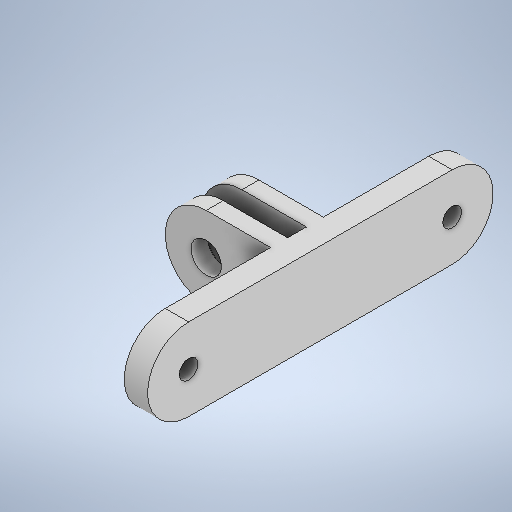
# Autodesk Inventor part: support_realsense
Saved by Autodesk Inventor 2025.2 (Build 292293000, 293)
## iProperties
Created: 2025-05-11
Part Number: support_realsense
Material: Générique
Document SubType Name: Modeling
Designer: enezl
Density: 1 g/cm^3
Appearance: Par défaut
Author: enezl
Autodesk Inventor part; units mm, degrees
ref_plane "YZ Plane" through (0, 0, 0) normal (1, 0, 0) x (0, 1, 0)
ref_plane "XZ Plane" through (0, 0, 0) normal (0, 1, 0) x (-1, 0, 0)
ref_plane "XY Plane" through (0, 0, 0) normal (0, 0, 1) x (1, 0, 0)
sketch "Esquisse1" plane through (0, 0, 0) normal (1, 0, 0) x (0, 1, 0)
  line L0 (0, 22.5) -> (0, -22.5) construction
  line L1 (-7, 22.5) -> (-7, -22.5)
  line L2 (7, -22.5) -> (7, 22.5)
  arc A0 (7, 22.5) -> (-7, 22.5) centre (0, 22.5) ccw
  arc A1 (-7, -22.5) -> (7, -22.5) centre (0, -22.5) ccw
  circle A2 centre (0, 22.5) radius 1.6
  circle A3 centre (0, -22.5) radius 1.6
  point P0 (0, 0)
  dimension "d0" = 45
  dimension "d1" = 3.2
  dimension "d2" = 14
  constraints: 8 end point, 4 centre point, 4 point on circle, 4 tangent, 2 coincident, 1 equal radius, 1 midpoint, 1 parallel, 1 vertical
  measures "d0" distance of L0.start L0.end
  measures "d1" diameter of A2
  measures "d2" distance between parallel lines of L1 L2
extrude "Extrusion1" add sketch "Esquisse1" along normal blind 4
sketch "Esquisse2" plane through (0, 7, 22.5) normal (0, 1, 0) x (1, 0, 0)
  line L0 (0, 51.1) -> (0, 0)
  line L1 (-18, 24.1) -> (0, 24.1)
  line L2 (0, 24.1) -> (0, 27)
  line L3 (0, 27) -> (-18, 27)
  line L4 (-18, 27) -> (-18, 24.1)
  line L5 (-18, 24.1) -> (0, 27) construction
  line L6 (0, 24.1) -> (-18, 27) construction
  line L7 (-18, 18) -> (0, 18)
  line L8 (0, 18) -> (0, 20.9)
  line L9 (0, 20.9) -> (-18, 20.9)
  line L10 (-18, 20.9) -> (-18, 18)
  line L11 (-18, 18) -> (0, 20.9) construction
  line L12 (0, 18) -> (-18, 20.9) construction
  line L13 (0, 18) -> (0, 27) construction
  line L14 (0, 45) -> (0, 0) construction
  point P0 (0, 22.5)
  point P1 (-9, 25.55)
  point P2 (-9, 19.45)
  point P3 (0, 25.55)
  point P4 (0, 22.5)
  point P5 (0, 24.1)
  point P6 (0, 18)
  point P7 (0, 20.9)
  dimension "d6" = 2.9
  dimension "d7" = 18
  dimension "d10" = 3.2
  constraints: 28 end point, 7 midpoint, 4 parallel, 2 collinear, 2 equal length, 2 horizontal, 1 perpendicular, 1 point on line, 2 other
  measures "d6" distance of L3.end L1.start
  measures "d7" distance of L2.end L3.end
  measures "d10" distance between parallel lines of L1 L9
extrude "Extrusion2" add sketch "Esquisse2" against normal up to surface (14 mm away)
sketch "Esquisse3" plane through (-18, 7, 4.5) normal (0, 0, 1) x (1, 0, 0)
  arc A0 (7, 0) -> (7, -14) centre (7, -7) ccw
  line L0 (0, 0) -> (18, 0) construction
  line L1 (7, 0) -> (18, 0)
  line L2 (18, -14) -> (7, -14)
  line L3 (18, 0) -> (18, 5)
  line L4 (18, 5) -> (-5, 5)
  line L5 (-5, 5) -> (-5, -19)
  line L6 (-5, -19) -> (18, -19)
  line L7 (18, -19) -> (18, -14)
  line L8 (18, 0) -> (18, -14) projected
  line L9 (0, 0) -> (0, -14) construction
  line L10 (0, -7) -> (-5, -7) construction
  circle A1 centre (7, -7) radius 2.6
  point P0 (18, -7)
  dimension "d11" = 14
  dimension "d12" = 5
  dimension "d16" = 5.2
  constraints: 16 end point, 4 perpendicular, 4 tangent, 2 centre point, 2 equal length, 2 midpoint, 2 point on circle, 1 coincident, 1 collinear, 1 horizontal, 1 parallel, 1 point on line, 1 vertical
  measures "d11" diameter of A0
  measures "d12" distance between parallel lines of L0 L4
  measures "d16" diameter of A1
extrude "Extrusion3" cut sketch "Esquisse3" against normal through all contours A0 L2 L7 L6 L5 L4 L3 L1 | A1
